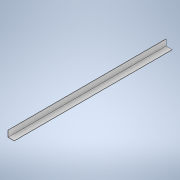
# Autodesk Inventor part: C_358_40_2
Saved by Autodesk Inventor 2020 (Build 240168000, 168)
## iProperties
Created: 2022-03-28
Part Number: C_358_40_2
Material: Genérico
Document SubType Name: Modeling
Designer: aarco
Density: 1 g/cm^3
Appearance: Valor por defecto
Author: aarco
Autodesk Inventor part; units mm, degrees
ref_plane "YZ Plane" through (0, 0, 0) normal (1, 0, 0) x (0, 1, 0)
ref_plane "XZ Plane" through (0, 0, 0) normal (0, 1, 0) x (-1, 0, 0)
ref_plane "XY Plane" through (0, 0, 0) normal (0, 0, 1) x (1, 0, 0)
sketch "Boceto1" plane through (0, 0, 0) normal (0, 0, 1) x (1, 0, 0)
  line L0 (-20, 20) -> (20, 20)
  line L1 (20, 20) -> (20, -20)
  line L2 (20, -20) -> (-20, -20)
  line L3 (-20, -20) -> (-20, 20)
  line L4 (-20, 20) -> (20, -20) construction
  line L5 (-18, 18) -> (18, 18)
  line L6 (18, 18) -> (18, -18)
  line L7 (18, -18) -> (-18, -18)
  line L8 (-18, -18) -> (-18, 18)
  line L9 (-18, 0) -> (-20, 0) construction
  line L10 (0, 18) -> (0, 20) construction
  line L11 (18, 0) -> (20, 0) construction
  line L12 (0, -18) -> (0, -20) construction
  line L13 (-18, 18) -> (-18, 20)
  line L14 (18, -18) -> (20, -18)
  point P0 (0, 0)
  point P1 (0, 0)
  dimension "d0" = 40
  dimension "d1" = 2
  dimension "d4" = 40
  constraints: 30 end point, 9 midpoint, 8 perpendicular, 4 parallel, 4 point on line, 2 horizontal, 1 coincident
  measures "d0" distance of L2.end L0.start
  measures "d1" distance of L10.start L10.end
  measures "d4" distance of L1.end L2.end
extrude "Extrusión1" add sketch "Boceto1" along normal blind 992 contours L0 L13 L8 L7 L14 L1 L2 L3
